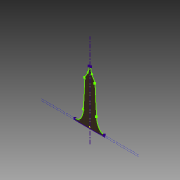
# Autodesk Inventor part: Bottom Plate v2
Saved by Autodesk Inventor 2013 SP1 (Build 170176100, 176)
## iProperties
Created: 2013-02-28
Part Number: Bottom Plate v2
Material: Wood (Cherry)
Document SubType Name: Modeling
Designer: fixer
Mass: 59.0239 g
Surface Area: 779.579 cm^2
Volume: 118.048 cm^3
Density: 0.5 g/cm^3
Author: fixer
Autodesk Inventor part; units mm, degrees
ref_plane "YZ Plane" through (0, 0, 0) normal (1, 0, 0) x (0, 1, 0)
ref_plane "XZ Plane" through (0, 0, 0) normal (0, 1, 0) x (-1, 0, 0)
ref_plane "XY Plane" through (0, 0, 0) normal (0, 0, 1) x (1, 0, 0)
sketch "Sketch1" plane through (0, 0, 0) normal (0, 0, 1) x (1, 0, 0)
  line L0 (76.2, -12.7) -> (381, -12.7) construction
  line L1 (-76.2, -12.7) -> (-381, -12.7) construction
  line L2 (-76.2, 0) -> (-381, 0) construction
  line L3 (76.2, 0) -> (381, 0) construction
  line L4 (0, -116.2267) -> (0, 608.4603)
  line L5 (0, -12.7) -> (-114.3, -12.7)
  line L6 (-114.3, -12.7) -> (-114.3, 0)
  line L7 (0, 406.4) -> (-6.35, 406.4)
  line L8 (-39.0138, 312.42) -> (-50.5988, 93.6374)
  line L9 (39.0138, 312.42) -> (50.5988, 93.6374)
  line L10 (0, 406.4) -> (6.35, 406.4)
  line L11 (0, -12.7) -> (114.3, -12.7)
  line L12 (114.3, -12.7) -> (114.3, 0)
  spline S0 degree 4 poles (-6.35, 406.4) (-6.35, 374.2572) (-17.7644, 366.5849) (-7.7511, 356.5096) (-38.295, 325.9934) (-39.0138, 312.42) knots 0 0 0 0 0 0.493995 1 1 1 1 1
  line L13 (-6.35, 450.2792) -> (-6.35, 362.5208) construction
  arc A0 (-8.8336, 371.6535) -> (-8.8336, 441.1465) centre (-250.6544, 406.4) ccw construction
  spline S1 degree 4 poles (6.35, 406.4) (6.35, 374.2572) (17.7644, 366.5849) (7.7511, 356.5096) (38.295, 325.9934) (39.0138, 312.42) knots 0 0 0 0 0 0.493995 1 1 1 1 1
  line L14 (6.35, 450.2792) -> (6.35, 362.5208) construction
  arc A1 (8.8336, 441.1465) -> (8.8336, 371.6535) centre (250.6544, 406.4) ccw construction
  line L15 (-11.4872, 368.6935) -> (-18.361, 349.9023) construction
  arc A2 (-18.0599, 351.9719) -> (-12.5926, 366.9181) centre (-84.5642, 384.7721) ccw construction
  line L16 (11.4872, 368.6935) -> (18.361, 349.9023) construction
  arc A3 (12.5926, 366.9181) -> (18.0599, 351.9719) centre (84.5642, 384.7721) ccw construction
  spline S2 degree 3 poles (-50.5988, 93.6374) (-52.7393, 53.2143) (-67.314, 0) (-114.3, 0) knots 0 0 0 0 1 1 1 1
  line L17 (-100.9407, 0) -> (-127.6593, 0) construction
  arc A4 (-124.8332, 0.8979) -> (-103.7668, 0.8979) centre (-114.3, 62.2299) ccw construction
  spline S3 degree 3 poles (50.5988, 93.6374) (52.7393, 53.2143) (67.314, 0) (114.3, 0) knots 0 0 0 0 1 1 1 1
  line L18 (100.9407, 0) -> (127.6593, 0) construction
  arc A5 (103.7668, 0.8979) -> (124.8332, 0.8979) centre (114.3, 62.2299) ccw construction
  point P0 (0, 0)
  point P1 (-14.9241, 359.2979)
  point P2 (14.9241, 359.2979)
  dimension "d0" = 6.35
  dimension "d3" = 114.3
  dimension "d4" = 419.1
  dimension "d5" = 0.6
  dimension "d6" = 0.6
  dimension "d7" = 93.98
  constraints: 38 end point, 15 symmetric about line, 10 midpoint, 9 horizontal, 6 centre point, 6 point on circle, 5 point on line, 4 vertical, 2 perpendicular, 25 other
  measures "d0" distance of L7.start L7.end
  measures "d3" distance of L5.start L11.end
  measures "d4" distance between parallel lines of L11 L10
  measures "d7" distance from line of L9.start L10
extrude "Extrusion1" add sketch "Sketch1" against normal blind 3.175
equation "\"d6\" = d5"
body "Solid1"
